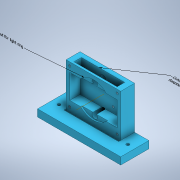
# Autodesk Inventor part: 2020PiZeroCameraLightRingMount
Saved by Autodesk Inventor 2020.2 (Build 242310000, 310)
## iProperties
Created: 2019-10-10
Part Number: 2020PiZeroCameraLightRingMount
Material: PC/ABS Plastic
Document SubType Name: Modeling
Designer: steele
Density: 0.357273 g/cm^3
Appearance: Turquoise
Author: steele
Autodesk Inventor part; units mm, degrees
ref_plane "YZ Plane" through (0, 0, 0) normal (1, 0, 0) x (0, 1, 0)
ref_plane "XZ Plane" through (0, 0, 0) normal (0, 1, 0) x (-1, 0, 0)
ref_plane "XY Plane" through (0, 0, 0) normal (0, 0, 1) x (1, 0, 0)
sketch "Sketch1" plane through (0, 0, 0) normal (0, 0, 1) x (1, 0, 0)
  line L0 (-48.5775, -37.85) -> (48.5775, -37.85)
  line L1 (48.5775, -37.85) -> (48.5775, 37.85)
  line L2 (48.5775, 37.85) -> (-48.5775, 37.85)
  line L3 (-48.5775, 37.85) -> (-48.5775, -37.85)
  line L4 (-48.5775, -37.85) -> (48.5775, 37.85) construction
  line L5 (48.5775, -37.85) -> (-48.5775, 37.85) construction
  point P0 (0, 0)
  dimension "majorPartWidth" = 97.155
  dimension "majorPartHeight" = 75.7
  constraints: 12 end point, 2 midpoint, 2 parallel, 1 horizontal, 1 perpendicular
  measures "majorPartWidth" distance of L0.start L0.end
  measures "majorPartHeight" distance of L1.end L0.end
extrude "Extrusion1" add sketch "Sketch1" against normal blind 24.725
sketch "Sketch2" plane through (0, 0, 0) normal (0, 0, 1) x (1, 0, 0)
  line L0 (-42.2275, -21.59) -> (42.2275, -21.59)
  line L1 (42.2275, -21.59) -> (42.2275, 21.59)
  line L2 (42.2275, 21.59) -> (-42.2275, 21.59)
  line L3 (-42.2275, 21.59) -> (-42.2275, -21.59)
  line L4 (-42.2275, -21.59) -> (42.2275, 21.59) construction
  line L5 (42.2275, -21.59) -> (-42.2275, 21.59) construction
  point P0 (0, 0)
  dimension "holeForPiCaseWidth" = 84.455
  dimension "holeForPiCaseHeight" = 43.18
  constraints: 12 end point, 2 midpoint, 2 parallel, 1 horizontal, 1 perpendicular
  measures "holeForPiCaseWidth" distance of L0.start L0.end
  measures "holeForPiCaseHeight" distance of L1.end L0.end
extrude "Extrusion2" cut sketch "Sketch2" against normal blind 18.375
sketch "Sketch3" plane through (0, 0, 0) normal (0, 0, 1) x (1, 0, 0)
  circle A0 centre (0, 0) radius 31.5
  circle A1 centre (0, 0) radius 18.5
  dimension "lightRingHoleExteriorDiam" = 63
  dimension "lightRingHoleInteriorDiam" = 37
  constraints: 2 centre point, 2 coincident
  measures "lightRingHoleExteriorDiam" diameter of A0
  measures "lightRingHoleInteriorDiam" diameter of A1
extrude "Extrusion3" cut sketch "Sketch3" against normal blind 2.5
sketch "Sketch4" plane through (0, 0, -2.5) normal (0, 0, 1) x (1, 0, 0)
  circle A0 centre (0, 0) radius 25.4466 construction
  circle A1 centre (0, 25.4466) radius 5
  circle A2 centre (0, -25.4466) radius 5
  dimension "holeForLightRingWires" = 10
  dimension "d13" = 10
  constraints: 3 centre point, 2 point on circle, 1 coincident
  measures "holeForLightRingWires" diameter of A1
  measures "d13" diameter of A2
extrude "Extrusion4" cut sketch "Sketch4" against normal through all
sketch "Sketch6" plane through (-48.5775, -37.85, 0) normal (0, -1, 0) x (1, 0, 0)
  line L0 (0, -24.725) -> (97.155, -24.725) projected
  line L1 (0, -24.725) -> (97.155, -24.725)
  line L2 (97.155, -24.725) -> (97.155, 25.4)
  line L3 (97.155, 25.4) -> (0, 25.4)
  line L4 (0, 25.4) -> (0, -24.725)
  point P0 (48.5775, 0)
  dimension "baseWidth" = 97.155
  dimension "baseDepth" = 50.125
  constraints: 8 end point, 2 parallel, 1 horizontal, 1 perpendicular
  measures "baseWidth" distance of L2.end L3.end
  measures "baseDepth" distance of L1.end L2.end
extrude "Extrusion6" add sketch "Sketch6" along normal blind 12.7
sketch "Sketch7" plane through (-48.5775, 37.85, 0) normal (0, 1, 0) x (1, 0, 0)
  line L0 (97.155, 0) -> (0, 0) construction
  line L1 (0, 0) -> (0, 24.725) construction
  line L2 (10.16, 3.77) -> (86.995, 3.77)
  line L3 (86.995, 3.77) -> (86.995, 17.105)
  line L4 (86.995, 17.105) -> (10.16, 17.105)
  line L5 (10.16, 17.105) -> (10.16, 3.77)
  line L6 (10.16, 3.77) -> (86.995, 17.105) construction
  line L7 (86.995, 3.77) -> (10.16, 17.105) construction
  line L8 (45.3952, 18.375) -> (45.3952, 2.5) projected
  point P0 (48.5775, 0)
  point P1 (48.5775, 10.4375)
  dimension "y" = 10.4375
  dimension "Y" = 48.5775
  dimension "piWireDepth" = 13.335
  dimension "piWireWidth" = 76.835
  constraints: 12 end point, 2 midpoint, 2 parallel, 2 perpendicular
  measures "y" distance from line of point (48.577, 10.438) L0
  measures "Y" distance from line of point (48.577, 10.438) L1
  measures "piWireDepth" distance of L4.end L2.start
  measures "piWireWidth" distance of L3.end L4.end
extrude "Extrusion7" cut sketch "Sketch7" against normal up to next
sketch "Sketch8" plane through (-48.5775, 37.85, -24.725) normal (-1, 0, 0) x (0, 0, 1)
  line L0 (24.725, -75.7) -> (24.725, 0) projected
  line L1 (24.725, -75.7) -> (28.535, -75.7)
  line L2 (28.535, -75.7) -> (28.535, -78.24)
  line L3 (28.535, -78.24) -> (24.725, -78.24)
  line L4 (24.725, -78.24) -> (24.725, -75.7)
  point P0 (24.725, -37.85)
  dimension "d30" = 3.81
  dimension "d31" = 2.54
  constraints: 8 end point, 2 parallel, 1 horizontal, 1 perpendicular
  measures "d30" distance of L2.end L3.end
  measures "d31" distance of L1.end L2.end
extrude "Extrusion8" cut sketch "Sketch8" against normal through all
sketch "Sketch9" plane through (0, 0, 0) normal (0, 0, 1) x (1, 0, 0)
  point P0 (-42.2275, 31.5)
  point P1 (42.2275, 31.5)
  point P2 (42.2275, -31.5)
  point P3 (-42.2275, -31.5)
hole "Hole1" at (-42.2275, 31.5, 0) at (42.2275, 31.5, 0) at (42.2275, -31.5, 0) at (-42.2275, -31.5, 0) direction (0, 0, -1) diameter 3.9624 depth 14.986 tip angle 120 thread size "10-32 UNF" class "2B" standard "ANSI Unified Screw Threads"
sketch "Sketch10" plane through (0, 0, -24.725) normal (0, 0, -1) x (-1, 0, 0)
  point P0 (-39.0525, 23.7022)
  point P1 (-16.8275, 23.7022)
  point P2 (-16.8275, -11.2228)
  point P3 (-39.0525, -11.2228)
hole "Hole3" at (39.0525, 23.7022, -24.725) at (16.8275, 23.7022, -24.725) at (16.8275, -11.2228, -24.725) at (39.0525, -11.2228, -24.725) direction (0, 0, 1) diameter 3.9624 depth 11.9507 tip angle 120 thread size "10-32 UNF" class "2B" standard "ANSI Unified Screw Threads"
sketch "Sketch11" plane through (48.5775, 37.85, 0) normal (1, 0, 0) x (0, 0, -1)
  line L0 (-25.4, -75.7) -> (-25.4, -88.4) projected
  line L1 (24.725, 0) -> (24.725, -88.4) projected
  line L2 (-25.4, -88.4) -> (24.725, -88.4)
  line L3 (24.725, -88.4) -> (24.725, -75.7)
  line L4 (24.725, -75.7) -> (-25.4, -75.7)
  line L5 (-25.4, -75.7) -> (-25.4, -88.4)
  point P0 (0, -37.85)
  dimension "d50" = 12.7
  constraints: 8 end point, 2 parallel, 1 horizontal, 1 perpendicular, 1 point on line
  measures "d50" distance of L3.end L2.end
extrude "Extrusion9" add sketch "Sketch11" along normal blind 25.4
sketch "Sketch12" plane through (-48.5775, 37.85, -24.725) normal (-1, 0, 0) x (0, 0, 1)
  line L0 (50.125, -75.7) -> (50.125, -88.4) projected
  line L1 (50.125, -88.4) -> (0, -88.4) projected
  line L2 (50.125, -75.7) -> (0, -75.7)
  line L3 (0, -75.7) -> (0, -88.4)
  line L4 (0, -88.4) -> (50.125, -88.4)
  line L5 (50.125, -88.4) -> (50.125, -75.7)
  point P0 (24.725, -37.85)
  constraints: 8 end point, 2 parallel, 1 horizontal, 1 perpendicular
extrude "Extrusion10" add sketch "Sketch12" along normal blind 25.4
sketch "Sketch13" plane through (-48.5775, -37.85, 0) normal (0, 1, 0) x (1, 0, 0)
  line L0 (97.155, 0) -> (0, 0) projected
  line L1 (0, 0) -> (0, 24.725) projected
  line L2 (97.155, 0) -> (97.155, 24.725) projected
  point P0 (48.5775, 0)
  point P1 (109.855, 0)
  point P2 (-12.7, 0)
  dimension "d62" = 0
  dimension "d63" = 0
  dimension "d64" = 12.7
  dimension "d65" = 12.7
  measures "d62" distance from line of point (-12.7, 0) L0
  measures "d63" distance from line of L0 point (109.855, 0)
  measures "d64" distance from line of point (-12.7, 0) L1
  measures "d65" distance from line of point (109.855, 0) L2
hole "Hole5" at (61.2775, -37.85, 0) at (-61.2775, -37.85, 0) direction (0, -1, 0) diameter 5.1054 end through all clearance for "Socket Head Cap Screw" size "#10" standard "Ansi Unified Screw Threads"
sketch "Sketch14" plane through (-48.5775, -50.55, 0) normal (0, -1, 0) x (1, 0, 0)
  circle A0 centre (-12.7, 0) radius 2.5527 construction
  circle A1 centre (109.855, 0) radius 2.5527 construction
  line L0 (-12.7, 0) -> (109.855, 0) construction
  spline S0 degree 2 poles (30.5129, 11.4249) (30.5129, 10.5552) (29.8079, 9.1555) (29.2162, 8.7644) knots 0 0 0 1 2 2 2
  spline S1 degree 2 poles (29.2162, 8.7644) (28.7325, 8.4608) (27.7393, 8.255) (26.9674, 8.255) knots 0 0 0 1 2 2 2
  line L1 (26.9674, 8.255) -> (25.506, 8.255)
  line L2 (25.506, 8.255) -> (25.506, 14.605)
  line L3 (25.506, 14.605) -> (26.952, 14.605)
  spline S2 degree 2 poles (26.952, 14.605) (27.8474, 14.605) (28.8663, 14.3374) (29.2265, 14.1007) knots 0 0 0 1 2 2 2
  spline S3 degree 2 poles (29.2265, 14.1007) (29.8388, 13.6942) (30.5129, 12.3511) (30.5129, 11.4249) knots 0 0 0 1 2 2 2
  spline S4 degree 2 poles (29.633, 11.4351) (29.633, 12.1659) (29.1493, 13.2002) (28.6707, 13.4935) knots 0 0 0 1 2 2 2
  spline S5 degree 2 poles (28.6707, 13.4935) (28.3311, 13.6942) (27.5644, 13.8743) (26.9932, 13.8743) knots 0 0 0 1 2 2 2
  line L4 (26.9932, 13.8743) -> (26.3499, 13.8743)
  line L5 (26.3499, 13.8743) -> (26.3499, 8.9857)
  line L6 (26.3499, 8.9857) -> (26.9932, 8.9857)
  spline S6 degree 2 poles (26.9932, 8.9857) (27.5541, 8.9857) (28.4031, 9.1658) (28.7479, 9.4077) knots 0 0 0 1 2 2 2
  spline S7 degree 2 poles (28.7479, 9.4077) (29.1904, 9.7061) (29.633, 10.6941) (29.633, 11.4351) knots 0 0 0 1 2 2 2
  spline S8 degree 2 poles (33.4358, 8.1469) (32.2934, 8.1469) (31.0378, 9.4283) (31.0378, 10.6118) knots 0 0 0 1 2 2 2
  spline S9 degree 2 poles (31.0378, 10.6118) (31.0378, 11.7748) (32.2574, 13.1539) (33.2402, 13.1539) knots 0 0 0 1 2 2 2
  spline S10 degree 2 poles (33.2402, 13.1539) (33.6828, 13.1539) (34.3672, 12.8966) (34.6193, 12.6238) knots 0 0 0 1 2 2 2
  spline S11 degree 2 poles (34.6193, 12.6238) (34.8766, 12.3511) (35.1494, 11.5638) (35.1494, 10.9926) knots 0 0 0 1 2 2 2
  line L7 (35.1494, 10.9926) -> (35.1494, 10.5552)
  line L8 (35.1494, 10.5552) -> (31.8509, 10.5552)
  spline S12 degree 2 poles (31.8509, 10.5552) (31.8509, 9.7267) (32.6845, 8.8468) (33.4255, 8.8468) knots 0 0 0 1 2 2 2
  spline S13 degree 2 poles (33.4255, 8.8468) (33.6879, 8.8468) (34.1974, 8.9651) (34.4032, 9.0578) knots 0 0 0 1 2 2 2
  spline S14 degree 2 poles (34.4032, 9.0578) (34.6193, 9.1607) (34.9178, 9.3408) (35.0156, 9.4231) knots 0 0 0 1 2 2 2
  line L9 (35.0156, 9.4231) -> (35.0619, 9.4231)
  line L10 (35.0619, 9.4231) -> (35.0619, 8.5483)
  spline S15 degree 2 poles (35.0619, 8.5483) (34.9229, 8.4917) (34.501, 8.327) (34.3363, 8.2807) knots 0 0 0 1 2 2 2
  spline S16 degree 2 poles (34.3363, 8.2807) (34.1047, 8.2138) (33.724, 8.1469) (33.4358, 8.1469) knots 0 0 0 1 2 2 2
  spline S17 degree 2 poles (34.3672, 11.1676) (34.3569, 11.4918) (34.2231, 11.9652) (34.0945, 12.1247) knots 0 0 0 1 2 2 2
  spline S18 degree 2 poles (34.0945, 12.1247) (33.9555, 12.3048) (33.5181, 12.4952) (33.1939, 12.4952) knots 0 0 0 1 2 2 2
  spline S19 degree 2 poles (33.1939, 12.4952) (32.8749, 12.4952) (32.4272, 12.3048) (32.2419, 12.1195) knots 0 0 0 1 2 2 2
  spline S20 degree 2 poles (32.2419, 12.1195) (32.0618, 11.9291) (31.8766, 11.4712) (31.8509, 11.1676) knots 0 0 0 1 2 2 2
  line L11 (31.8509, 11.1676) -> (34.3672, 11.1676)
  spline S21 degree 2 poles (37.2489, 8.1418) (36.7703, 8.1418) (35.9418, 8.3991) (35.6691, 8.5432) knots 0 0 0 1 2 2 2
  line L12 (35.6691, 8.5432) -> (35.6691, 9.4437)
  line L13 (35.6691, 9.4437) -> (35.7103, 9.4437)
  spline S22 degree 2 poles (35.7103, 9.4437) (35.8132, 9.3614) (36.0911, 9.1658) (36.3226, 9.0578) knots 0 0 0 1 2 2 2
  spline S23 degree 2 poles (36.3226, 9.0578) (36.5233, 8.96) (37.0173, 8.8159) (37.2797, 8.8159) knots 0 0 0 1 2 2 2
  spline S24 degree 2 poles (37.2797, 8.8159) (37.4701, 8.8159) (37.9075, 8.9034) (38.0105, 8.9754) knots 0 0 0 1 2 2 2
  spline S25 degree 2 poles (38.0105, 8.9754) (38.1597, 9.0732) (38.2935, 9.2945) (38.2935, 9.5209) knots 0 0 0 1 2 2 2
  spline S26 degree 2 poles (38.2935, 9.5209) (38.2935, 9.8039) (37.9847, 10.0972) (37.5885, 10.195) knots 0 0 0 1 2 2 2
  spline S27 degree 2 poles (37.5885, 10.195) (37.4341, 10.231) (36.9401, 10.3339) (36.7291, 10.3905) knots 0 0 0 1 2 2 2
  spline S28 degree 2 poles (36.7291, 10.3905) (36.1837, 10.5501) (35.6897, 11.2087) (35.6897, 11.677) knots 0 0 0 1 2 2 2
  spline S29 degree 2 poles (35.6897, 11.677) (35.6897, 12.3254) (36.6622, 13.1333) (37.465, 13.1333) knots 0 0 0 1 2 2 2
  spline S30 degree 2 poles (37.465, 13.1333) (37.8612, 13.1333) (38.664, 12.9377) (38.9367, 12.7885) knots 0 0 0 1 2 2 2
  line L14 (38.9367, 12.7885) -> (38.9367, 11.9291)
  line L15 (38.9367, 11.9291) -> (38.8956, 11.9291)
  spline S31 degree 2 poles (38.8956, 11.9291) (38.5868, 12.1762) (37.8355, 12.4592) (37.4496, 12.4592) knots 0 0 0 1 2 2 2
  spline S32 degree 2 poles (37.4496, 12.4592) (37.0533, 12.4592) (36.5079, 12.1247) (36.5079, 11.7902) knots 0 0 0 1 2 2 2
  spline S33 degree 2 poles (36.5079, 11.7902) (36.5079, 11.4866) (36.8321, 11.1933) (37.1923, 11.1007) knots 0 0 0 1 2 2 2
  spline S34 degree 2 poles (37.1923, 11.1007) (37.3672, 11.0544) (37.8098, 10.9617) (38.0516, 10.9051) knots 0 0 0 1 2 2 2
  spline S35 degree 2 poles (38.0516, 10.9051) (38.5765, 10.7713) (39.1117, 10.159) (39.1117, 9.6289) knots 0 0 0 1 2 2 2
  spline S36 degree 2 poles (39.1117, 9.6289) (39.1117, 9.3202) (38.8698, 8.7747) (38.6331, 8.574) knots 0 0 0 1 2 2 2
  spline S37 degree 2 poles (38.6331, 8.574) (38.381, 8.3631) (37.7377, 8.1418) (37.2489, 8.1418) knots 0 0 0 1 2 2 2
  line L16 (40.676, 8.255) -> (39.8733, 8.255)
  line L17 (39.8733, 8.255) -> (39.8733, 13.0201)
  line L18 (39.8733, 13.0201) -> (40.676, 13.0201)
  line L19 (40.676, 13.0201) -> (40.676, 8.255)
  line L20 (40.7326, 13.8125) -> (39.8218, 13.8125)
  line L21 (39.8218, 13.8125) -> (39.8218, 14.6462)
  line L22 (39.8218, 14.6462) -> (40.7326, 14.6462)
  line L23 (40.7326, 14.6462) -> (40.7326, 13.8125)
  spline S38 degree 2 poles (42.0242, 7.4934) (42.1066, 7.4574) (42.4205, 7.3442) (42.6212, 7.2979) knots 0 0 0 1 2 2 2
  spline S39 degree 2 poles (42.6212, 7.2979) (42.8424, 7.2413) (43.2181, 7.1744) (43.4394, 7.1744) knots 0 0 0 1 2 2 2
  spline S40 degree 2 poles (43.4394, 7.1744) (43.8099, 7.1744) (44.3244, 7.3699) (44.4685, 7.5449) knots 0 0 0 1 2 2 2
  spline S41 degree 2 poles (44.4685, 7.5449) (44.6075, 7.7198) (44.7155, 8.1778) (44.7155, 8.4711) knots 0 0 0 1 2 2 2
  line L24 (44.7155, 8.4711) -> (44.7155, 8.8879)
  spline S42 degree 2 poles (44.7155, 8.8879) (44.3913, 8.6049) (43.7687, 8.3373) (43.3004, 8.3373) knots 0 0 0 1 2 2 2
  spline S43 degree 2 poles (43.3004, 8.3373) (42.4874, 8.3373) (41.5251, 9.5466) (41.5251, 10.6838) knots 0 0 0 1 2 2 2
  spline S44 degree 2 poles (41.5251, 10.6838) (41.5251, 11.2756) (41.8596, 12.1916) (42.1374, 12.5158) knots 0 0 0 1 2 2 2
  spline S45 degree 2 poles (42.1374, 12.5158) (42.405, 12.8194) (43.1409, 13.1539) (43.532, 13.1539) knots 0 0 0 1 2 2 2
  spline S46 degree 2 poles (43.532, 13.1539) (43.9025, 13.1539) (44.4428, 12.9789) (44.7155, 12.8194) knots 0 0 0 1 2 2 2
  line L25 (44.7155, 12.8194) -> (44.7618, 13.0201)
  line L26 (44.7618, 13.0201) -> (45.5183, 13.0201)
  line L27 (45.5183, 13.0201) -> (45.5183, 8.8005)
  spline S47 degree 2 poles (45.5183, 8.8005) (45.5183, 7.586) (44.4634, 6.4539) (43.3776, 6.4539) knots 0 0 0 1 2 2 2
  spline S48 degree 2 poles (43.3776, 6.4539) (43.0277, 6.4539) (42.297, 6.5672) (41.9831, 6.6598) knots 0 0 0 1 2 2 2
  line L28 (41.9831, 6.6598) -> (41.9831, 7.4934)
  line L29 (41.9831, 7.4934) -> (42.0242, 7.4934)
  line L30 (44.7155, 9.5466) -> (44.7155, 12.1659)
  spline S49 degree 2 poles (44.7155, 12.1659) (44.4171, 12.3099) (43.9128, 12.4334) (43.6606, 12.4334) knots 0 0 0 1 2 2 2
  spline S50 degree 2 poles (43.6606, 12.4334) (43.0534, 12.4334) (42.3536, 11.5381) (42.3536, 10.6993) knots 0 0 0 1 2 2 2
  spline S51 degree 2 poles (42.3536, 10.6993) (42.3536, 9.9068) (42.8836, 9.0783) (43.4805, 9.0783) knots 0 0 0 1 2 2 2
  spline S52 degree 2 poles (43.4805, 9.0783) (43.7944, 9.0783) (44.4531, 9.3253) (44.7155, 9.5466) knots 0 0 0 1 2 2 2
  line L31 (50.4223, 8.255) -> (49.6195, 8.255)
  line L32 (49.6195, 8.255) -> (49.6195, 10.972)
  spline S53 degree 2 poles (49.6195, 10.972) (49.6195, 11.3014) (49.5578, 11.8674) (49.4652, 12.0372) knots 0 0 0 1 2 2 2
  spline S54 degree 2 poles (49.4652, 12.0372) (49.3674, 12.2173) (49.0175, 12.3923) (48.719, 12.3923) knots 0 0 0 1 2 2 2
  spline S55 degree 2 poles (48.719, 12.3923) (48.4206, 12.3923) (47.7876, 12.0732) (47.484, 11.8159) knots 0 0 0 1 2 2 2
  line L33 (47.484, 11.8159) -> (47.484, 8.255)
  line L34 (47.484, 8.255) -> (46.6812, 8.255)
  line L35 (46.6812, 8.255) -> (46.6812, 13.0201)
  line L36 (46.6812, 13.0201) -> (47.484, 13.0201)
  line L37 (47.484, 13.0201) -> (47.484, 12.49)
  spline S56 degree 2 poles (47.484, 12.49) (47.8442, 12.8142) (48.5389, 13.1539) (48.93, 13.1539) knots 0 0 0 1 2 2 2
  spline S57 degree 2 poles (48.93, 13.1539) (49.6298, 13.1539) (50.4223, 12.2276) (50.4223, 11.3477) knots 0 0 0 1 2 2 2
  line L38 (50.4223, 11.3477) -> (50.4223, 8.255)
  spline S58 degree 2 poles (53.6179, 8.1469) (52.4755, 8.1469) (51.2199, 9.4283) (51.2199, 10.6118) knots 0 0 0 1 2 2 2
  spline S59 degree 2 poles (51.2199, 10.6118) (51.2199, 11.7748) (52.4395, 13.1539) (53.4223, 13.1539) knots 0 0 0 1 2 2 2
  spline S60 degree 2 poles (53.4223, 13.1539) (53.8649, 13.1539) (54.5493, 12.8966) (54.8014, 12.6238) knots 0 0 0 1 2 2 2
  spline S61 degree 2 poles (54.8014, 12.6238) (55.0587, 12.3511) (55.3314, 11.5638) (55.3314, 10.9926) knots 0 0 0 1 2 2 2
  line L39 (55.3314, 10.9926) -> (55.3314, 10.5552)
  line L40 (55.3314, 10.5552) -> (52.0329, 10.5552)
  spline S62 degree 2 poles (52.0329, 10.5552) (52.0329, 9.7267) (52.8666, 8.8468) (53.6076, 8.8468) knots 0 0 0 1 2 2 2
  spline S63 degree 2 poles (53.6076, 8.8468) (53.87, 8.8468) (54.3795, 8.9651) (54.5853, 9.0578) knots 0 0 0 1 2 2 2
  spline S64 degree 2 poles (54.5853, 9.0578) (54.8014, 9.1607) (55.0999, 9.3408) (55.1977, 9.4231) knots 0 0 0 1 2 2 2
  line L41 (55.1977, 9.4231) -> (55.244, 9.4231)
  line L42 (55.244, 9.4231) -> (55.244, 8.5483)
  spline S65 degree 2 poles (55.244, 8.5483) (55.105, 8.4917) (54.6831, 8.327) (54.5184, 8.2807) knots 0 0 0 1 2 2 2
  spline S66 degree 2 poles (54.5184, 8.2807) (54.2868, 8.2138) (53.906, 8.1469) (53.6179, 8.1469) knots 0 0 0 1 2 2 2
  spline S67 degree 2 poles (54.5493, 11.1676) (54.539, 11.4918) (54.4052, 11.9652) (54.2765, 12.1247) knots 0 0 0 1 2 2 2
  spline S68 degree 2 poles (54.2765, 12.1247) (54.1376, 12.3048) (53.7002, 12.4952) (53.376, 12.4952) knots 0 0 0 1 2 2 2
  spline S69 degree 2 poles (53.376, 12.4952) (53.057, 12.4952) (52.6093, 12.3048) (52.424, 12.1195) knots 0 0 0 1 2 2 2
  spline S70 degree 2 poles (52.424, 12.1195) (52.2439, 11.9291) (52.0587, 11.4712) (52.0329, 11.1676) knots 0 0 0 1 2 2 2
  line L43 (52.0329, 11.1676) -> (54.5493, 11.1676)
  line L44 (59.8084, 8.255) -> (59.0056, 8.255)
  line L45 (59.0056, 8.255) -> (59.0056, 8.7387)
  spline S71 degree 2 poles (59.0056, 8.7387) (58.8203, 8.5843) (58.5476, 8.3785) (58.3624, 8.291) knots 0 0 0 1 2 2 2
  spline S72 degree 2 poles (58.3624, 8.291) (58.1926, 8.2087) (57.8272, 8.1212) (57.5853, 8.1212) knots 0 0 0 1 2 2 2
  spline S73 degree 2 poles (57.5853, 8.1212) (57.1943, 8.1212) (56.5356, 8.4454) (56.304, 8.7593) knots 0 0 0 1 2 2 2
  spline S74 degree 2 poles (56.304, 8.7593) (56.0725, 9.0732) (55.8152, 9.9994) (55.8152, 10.6015) knots 0 0 0 1 2 2 2
  spline S75 degree 2 poles (55.8152, 10.6015) (55.8152, 11.2293) (56.1394, 12.1453) (56.4224, 12.49) knots 0 0 0 1 2 2 2
  spline S76 degree 2 poles (56.4224, 12.49) (56.6848, 12.7988) (57.4207, 13.1539) (57.8272, 13.1539) knots 0 0 0 1 2 2 2
  spline S77 degree 2 poles (57.8272, 13.1539) (58.1823, 13.1539) (58.7123, 12.9943) (59.0056, 12.8297) knots 0 0 0 1 2 2 2
  line L46 (59.0056, 12.8297) -> (59.0056, 14.888)
  line L47 (59.0056, 14.888) -> (59.8084, 14.888)
  line L48 (59.8084, 14.888) -> (59.8084, 8.255)
  line L49 (59.0056, 9.4128) -> (59.0056, 12.1659)
  spline S78 degree 2 poles (59.0056, 12.1659) (58.7071, 12.3099) (58.2337, 12.418) (57.961, 12.418) knots 0 0 0 1 2 2 2
  spline S79 degree 2 poles (57.961, 12.418) (57.3435, 12.418) (56.6436, 11.4918) (56.6436, 10.617) knots 0 0 0 1 2 2 2
  spline S80 degree 2 poles (56.6436, 10.617) (56.6436, 9.773) (57.1788, 8.8828) (57.7706, 8.8828) knots 0 0 0 1 2 2 2
  spline S81 degree 2 poles (57.7706, 8.8828) (58.0845, 8.8828) (58.7226, 9.171) (59.0056, 9.4128) knots 0 0 0 1 2 2 2
  spline S82 degree 2 poles (67.6918, 10.7147) (67.6918, 9.5466) (66.5597, 8.1212) (65.7055, 8.1212) knots 0 0 0 1 2 2 2
  spline S83 degree 2 poles (65.7055, 8.1212) (65.3196, 8.1212) (64.769, 8.3116) (64.5014, 8.4763) knots 0 0 0 1 2 2 2
  line L50 (64.5014, 8.4763) -> (64.4499, 8.255)
  line L51 (64.4499, 8.255) -> (63.6986, 8.255)
  line L52 (63.6986, 8.255) -> (63.6986, 14.888)
  line L53 (63.6986, 14.888) -> (64.5014, 14.888)
  line L54 (64.5014, 14.888) -> (64.5014, 12.5209)
  spline S84 degree 2 poles (64.5014, 12.5209) (64.805, 12.7937) (65.51, 13.1539) (65.9577, 13.1539) knots 0 0 0 1 2 2 2
  spline S85 degree 2 poles (65.9577, 13.1539) (66.7656, 13.1539) (67.6918, 11.8623) (67.6918, 10.7147) knots 0 0 0 1 2 2 2
  spline S86 degree 2 poles (66.8633, 10.653) (66.8633, 11.5072) (66.3436, 12.3923) (65.7673, 12.3923) knots 0 0 0 1 2 2 2
  spline S87 degree 2 poles (65.7673, 12.3923) (65.4431, 12.3923) (64.7741, 12.0835) (64.5014, 11.8468) knots 0 0 0 1 2 2 2
  line L55 (64.5014, 11.8468) -> (64.5014, 9.1144)
  spline S88 degree 2 poles (64.5014, 9.1144) (64.805, 8.9651) (65.2733, 8.8416) (65.5511, 8.8416) knots 0 0 0 1 2 2 2
  spline S89 degree 2 poles (65.5511, 8.8416) (66.1635, 8.8416) (66.8633, 9.7113) (66.8633, 10.653) knots 0 0 0 1 2 2 2
  line L56 (72.2665, 13.0201) -> (69.7039, 6.5003)
  line L57 (69.7039, 6.5003) -> (68.8445, 6.5003)
  line L58 (68.8445, 6.5003) -> (69.6987, 8.4866)
  line L59 (69.6987, 8.4866) -> (67.9697, 13.0201)
  line L60 (67.9697, 13.0201) -> (68.8342, 13.0201)
  line L61 (68.8342, 13.0201) -> (70.1361, 9.49)
  line L62 (70.1361, 9.49) -> (71.4329, 13.0201)
  line L63 (71.4329, 13.0201) -> (72.2665, 13.0201)
  line L64 (33.495, -2.3804) -> (32.3989, -2.3804)
  line L65 (32.3989, -2.3804) -> (30.392, 0.1463)
  line L66 (30.392, 0.1463) -> (29.4246, 0.1463)
  line L67 (29.4246, 0.1463) -> (29.4246, -2.3804)
  line L68 (29.4246, -2.3804) -> (28.5807, -2.3804)
  line L69 (28.5807, -2.3804) -> (28.5807, 3.9696)
  line L70 (28.5807, 3.9696) -> (30.217, 3.9696)
  spline S90 degree 2 poles (30.217, 3.9696) (30.7625, 3.9696) (31.4984, 3.8513) (31.8328, 3.6352) knots 0 0 0 1 2 2 2
  spline S91 degree 2 poles (31.8328, 3.6352) (32.1673, 3.419) (32.5533, 2.7449) (32.5533, 2.2458) knots 0 0 0 1 2 2 2
  spline S92 degree 2 poles (32.5533, 2.2458) (32.5533, 1.5511) (31.8431, 0.6094) (31.2359, 0.383) knots 0 0 0 1 2 2 2
  line L71 (31.2359, 0.383) -> (33.495, -2.3804)
  spline S93 degree 2 poles (31.6733, 2.1789) (31.6733, 2.4568) (31.4778, 2.8839) (31.2719, 3.0228) knots 0 0 0 1 2 2 2
  spline S94 degree 2 poles (31.2719, 3.0228) (31.0918, 3.1412) (30.6133, 3.2389) (30.2634, 3.2389) knots 0 0 0 1 2 2 2
  line L72 (30.2634, 3.2389) -> (29.4246, 3.2389)
  line L73 (29.4246, 3.2389) -> (29.4246, 0.8512)
  line L74 (29.4246, 0.8512) -> (30.1656, 0.8512)
  spline S95 degree 2 poles (30.1656, 0.8512) (30.5309, 0.8512) (31.1124, 0.9799) (31.3131, 1.1806) knots 0 0 0 1 2 2 2
  spline S96 degree 2 poles (31.3131, 1.1806) (31.4984, 1.3555) (31.6733, 1.8495) (31.6733, 2.1789) knots 0 0 0 1 2 2 2
  spline S97 degree 2 poles (37.8535, 0.0022) (37.8535, -1.202) (36.6957, -2.5142) (35.7283, -2.5142) knots 0 0 0 1 2 2 2
  spline S98 degree 2 poles (35.7283, -2.5142) (34.7351, -2.5142) (33.5979, -1.1608) (33.5979, 0.0022) knots 0 0 0 1 2 2 2
  spline S99 degree 2 poles (33.5979, 0.0022) (33.5979, 1.196) (34.7711, 2.5185) (35.7283, 2.5185) knots 0 0 0 1 2 2 2
  spline S100 degree 2 poles (35.7283, 2.5185) (36.6957, 2.5185) (37.8535, 1.2012) (37.8535, 0.0022) knots 0 0 0 1 2 2 2
  spline S101 degree 2 poles (37.025, 0.0022) (37.025, 0.9284) (36.3509, 1.829) (35.7283, 1.829) knots 0 0 0 1 2 2 2
  spline S102 degree 2 poles (35.7283, 1.829) (35.1056, 1.829) (34.4264, 0.9284) (34.4264, 0.0022) knots 0 0 0 1 2 2 2
  spline S103 degree 2 poles (34.4264, 0.0022) (34.4264, -0.8984) (35.1056, -1.8246) (35.7283, -1.8246) knots 0 0 0 1 2 2 2
  spline S104 degree 2 poles (35.7283, -1.8246) (36.3458, -1.8246) (37.025, -0.9138) (37.025, 0.0022) knots 0 0 0 1 2 2 2
  spline S105 degree 2 poles (42.67, 0.0794) (42.67, -1.0887) (41.538, -2.5142) (40.6837, -2.5142) knots 0 0 0 1 2 2 2
  spline S106 degree 2 poles (40.6837, -2.5142) (40.2978, -2.5142) (39.7472, -2.3238) (39.4796, -2.1591) knots 0 0 0 1 2 2 2
  line L75 (39.4796, -2.1591) -> (39.4281, -2.3804)
  line L76 (39.4281, -2.3804) -> (38.6769, -2.3804)
  line L77 (38.6769, -2.3804) -> (38.6769, 4.2527)
  line L78 (38.6769, 4.2527) -> (39.4796, 4.2527)
  line L79 (39.4796, 4.2527) -> (39.4796, 1.8856)
  spline S107 degree 2 poles (39.4796, 1.8856) (39.7832, 2.1583) (40.4882, 2.5185) (40.9359, 2.5185) knots 0 0 0 1 2 2 2
  spline S108 degree 2 poles (40.9359, 2.5185) (41.7438, 2.5185) (42.67, 1.2269) (42.67, 0.0794) knots 0 0 0 1 2 2 2
  spline S109 degree 2 poles (41.8416, 0.0176) (41.8416, 0.8718) (41.3218, 1.7569) (40.7455, 1.7569) knots 0 0 0 1 2 2 2
  spline S110 degree 2 poles (40.7455, 1.7569) (40.4213, 1.7569) (39.7523, 1.4482) (39.4796, 1.2115) knots 0 0 0 1 2 2 2
  line L80 (39.4796, 1.2115) -> (39.4796, -1.521)
  spline S111 degree 2 poles (39.4796, -1.521) (39.7832, -1.6702) (40.2515, -1.7937) (40.5294, -1.7937) knots 0 0 0 1 2 2 2
  spline S112 degree 2 poles (40.5294, -1.7937) (41.1417, -1.7937) (41.8416, -0.9241) (41.8416, 0.0176) knots 0 0 0 1 2 2 2
  spline S113 degree 2 poles (48.0629, -2.4936) (47.3734, -2.4936) (46.4059, -2.2054) (45.9788, -1.9996) knots 0 0 0 1 2 2 2
  line L81 (45.9788, -1.9996) -> (45.9788, -0.9395)
  line L82 (45.9788, -0.9395) -> (46.0406, -0.9395)
  spline S114 degree 2 poles (46.0406, -0.9395) (46.4574, -1.3306) (47.5123, -1.7629) (48.0012, -1.7629) knots 0 0 0 1 2 2 2
  spline S115 degree 2 poles (48.0012, -1.7629) (48.701, -1.7629) (49.4163, -1.1814) (49.4163, -0.7028) knots 0 0 0 1 2 2 2
  spline S116 degree 2 poles (49.4163, -0.7028) (49.4163, -0.322) (49.0406, 0.1514) (48.6341, 0.2698) knots 0 0 0 1 2 2 2
  spline S117 degree 2 poles (48.6341, 0.2698) (48.3408, 0.3521) (47.8519, 0.4653) (47.4866, 0.5579) knots 0 0 0 1 2 2 2
  spline S118 degree 2 poles (47.4866, 0.5579) (47.1572, 0.6454) (46.6375, 0.9078) (46.4368, 1.1188) knots 0 0 0 1 2 2 2
  spline S119 degree 2 poles (46.4368, 1.1188) (46.2413, 1.3298) (46.0251, 1.8959) (46.0251, 2.2664) knots 0 0 0 1 2 2 2
  spline S120 degree 2 poles (46.0251, 2.2664) (46.0251, 3.0382) (47.2293, 4.0828) (48.1607, 4.0828) knots 0 0 0 1 2 2 2
  spline S121 degree 2 poles (48.1607, 4.0828) (48.6959, 4.0828) (49.6427, 3.8719) (50.0492, 3.6712) knots 0 0 0 1 2 2 2
  line L83 (50.0492, 3.6712) -> (50.0492, 2.6626)
  line L84 (50.0492, 2.6626) -> (49.9875, 2.6626)
  spline S122 degree 2 poles (49.9875, 2.6626) (49.6839, 2.9405) (48.737, 3.3521) (48.2173, 3.3521) knots 0 0 0 1 2 2 2
  spline S123 degree 2 poles (48.2173, 3.3521) (47.6307, 3.3521) (46.9051, 2.8015) (46.9051, 2.3538) knots 0 0 0 1 2 2 2
  spline S124 degree 2 poles (46.9051, 2.3538) (46.9051, 1.9525) (47.3322, 1.4739) (47.7336, 1.3658) knots 0 0 0 1 2 2 2
  spline S125 degree 2 poles (47.7336, 1.3658) (48.0012, 1.2938) (48.7782, 1.1085) (49.0355, 1.0313) knots 0 0 0 1 2 2 2
  spline S126 degree 2 poles (49.0355, 1.0313) (49.689, 0.8307) (50.2962, 0.0228) (50.2962, -0.569) knots 0 0 0 1 2 2 2
  spline S127 degree 2 poles (50.2962, -0.569) (50.2962, -0.9447) (49.9926, -1.6651) (49.7199, -1.9172) knots 0 0 0 1 2 2 2
  spline S128 degree 2 poles (49.7199, -1.9172) (49.4163, -2.1951) (48.6444, -2.4936) (48.0629, -2.4936) knots 0 0 0 1 2 2 2
  spline S129 degree 2 poles (52.5347, -2.473) (51.8811, -2.473) (51.1453, -1.7268) (51.1453, -0.9189) knots 0 0 0 1 2 2 2
  line L85 (51.1453, -0.9189) -> (51.1453, 1.7209)
  line L86 (51.1453, 1.7209) -> (50.605, 1.7209)
  line L87 (50.605, 1.7209) -> (50.605, 2.3847)
  line L88 (50.605, 2.3847) -> (51.1453, 2.3847)
  line L89 (51.1453, 2.3847) -> (51.1453, 3.7535)
  line L90 (51.1453, 3.7535) -> (51.948, 3.7535)
  line L91 (51.948, 3.7535) -> (51.948, 2.3847)
  line L92 (51.948, 2.3847) -> (53.4249, 2.3847)
  line L93 (53.4249, 2.3847) -> (53.4249, 1.7209)
  line L94 (53.4249, 1.7209) -> (51.948, 1.7209)
  line L95 (51.948, 1.7209) -> (51.948, -0.5484)
  spline S130 degree 2 poles (51.948, -0.5484) (51.948, -0.9086) (51.9738, -1.3049) (52.0613, -1.4747) knots 0 0 0 1 2 2 2
  spline S131 degree 2 poles (52.0613, -1.4747) (52.1333, -1.6239) (52.4575, -1.7731) (52.7354, -1.7731) knots 0 0 0 1 2 2 2
  spline S132 degree 2 poles (52.7354, -1.7731) (52.9309, -1.7731) (53.2963, -1.6548) (53.3786, -1.6188) knots 0 0 0 1 2 2 2
  line L96 (53.3786, -1.6188) -> (53.4249, -1.6188)
  line L97 (53.4249, -1.6188) -> (53.4249, -2.3392)
  spline S133 degree 2 poles (53.4249, -2.3392) (53.1985, -2.4009) (52.7354, -2.473) (52.5347, -2.473) knots 0 0 0 1 2 2 2
  spline S134 degree 2 poles (56.0853, -2.4884) (54.9429, -2.4884) (53.6873, -1.2071) (53.6873, -0.0236) knots 0 0 0 1 2 2 2
  spline S135 degree 2 poles (53.6873, -0.0236) (53.6873, 1.1394) (54.9069, 2.5185) (55.8898, 2.5185) knots 0 0 0 1 2 2 2
  spline S136 degree 2 poles (55.8898, 2.5185) (56.3323, 2.5185) (57.0167, 2.2612) (57.2689, 1.9885) knots 0 0 0 1 2 2 2
  spline S137 degree 2 poles (57.2689, 1.9885) (57.5262, 1.7157) (57.7989, 0.9284) (57.7989, 0.3572) knots 0 0 0 1 2 2 2
  line L98 (57.7989, 0.3572) -> (57.7989, -0.0802)
  line L99 (57.7989, -0.0802) -> (54.5004, -0.0802)
  spline S138 degree 2 poles (54.5004, -0.0802) (54.5004, -0.9086) (55.334, -1.7886) (56.075, -1.7886) knots 0 0 0 1 2 2 2
  spline S139 degree 2 poles (56.075, -1.7886) (56.3375, -1.7886) (56.8469, -1.6702) (57.0527, -1.5776) knots 0 0 0 1 2 2 2
  spline S140 degree 2 poles (57.0527, -1.5776) (57.2689, -1.4747) (57.5673, -1.2946) (57.6651, -1.2122) knots 0 0 0 1 2 2 2
  line L100 (57.6651, -1.2122) -> (57.7114, -1.2122)
  line L101 (57.7114, -1.2122) -> (57.7114, -2.087)
  spline S141 degree 2 poles (57.7114, -2.087) (57.5725, -2.1437) (57.1505, -2.3083) (56.9858, -2.3546) knots 0 0 0 1 2 2 2
  spline S142 degree 2 poles (56.9858, -2.3546) (56.7543, -2.4215) (56.3735, -2.4884) (56.0853, -2.4884) knots 0 0 0 1 2 2 2
  spline S143 degree 2 poles (57.0167, 0.5322) (57.0064, 0.8564) (56.8726, 1.3298) (56.744, 1.4893) knots 0 0 0 1 2 2 2
  spline S144 degree 2 poles (56.744, 1.4893) (56.6051, 1.6694) (56.1677, 1.8598) (55.8435, 1.8598) knots 0 0 0 1 2 2 2
  spline S145 degree 2 poles (55.8435, 1.8598) (55.5244, 1.8598) (55.0767, 1.6694) (54.8915, 1.4842) knots 0 0 0 1 2 2 2
  spline S146 degree 2 poles (54.8915, 1.4842) (54.7114, 1.2938) (54.5261, 0.8358) (54.5004, 0.5322) knots 0 0 0 1 2 2 2
  line L102 (54.5004, 0.5322) -> (57.0167, 0.5322)
  spline S147 degree 2 poles (60.6806, -2.4884) (59.5382, -2.4884) (58.2826, -1.2071) (58.2826, -0.0236) knots 0 0 0 1 2 2 2
  spline S148 degree 2 poles (58.2826, -0.0236) (58.2826, 1.1394) (59.5022, 2.5185) (60.485, 2.5185) knots 0 0 0 1 2 2 2
  spline S149 degree 2 poles (60.485, 2.5185) (60.9276, 2.5185) (61.612, 2.2612) (61.8641, 1.9885) knots 0 0 0 1 2 2 2
  spline S150 degree 2 poles (61.8641, 1.9885) (62.1214, 1.7157) (62.3942, 0.9284) (62.3942, 0.3572) knots 0 0 0 1 2 2 2
  line L103 (62.3942, 0.3572) -> (62.3942, -0.0802)
  line L104 (62.3942, -0.0802) -> (59.0957, -0.0802)
  spline S151 degree 2 poles (59.0957, -0.0802) (59.0957, -0.9086) (59.9293, -1.7886) (60.6703, -1.7886) knots 0 0 0 1 2 2 2
  spline S152 degree 2 poles (60.6703, -1.7886) (60.9327, -1.7886) (61.4422, -1.6702) (61.648, -1.5776) knots 0 0 0 1 2 2 2
  spline S153 degree 2 poles (61.648, -1.5776) (61.8641, -1.4747) (62.1626, -1.2946) (62.2604, -1.2122) knots 0 0 0 1 2 2 2
  line L105 (62.2604, -1.2122) -> (62.3067, -1.2122)
  line L106 (62.3067, -1.2122) -> (62.3067, -2.087)
  spline S154 degree 2 poles (62.3067, -2.087) (62.1677, -2.1437) (61.7458, -2.3083) (61.5811, -2.3546) knots 0 0 0 1 2 2 2
  spline S155 degree 2 poles (61.5811, -2.3546) (61.3495, -2.4215) (60.9687, -2.4884) (60.6806, -2.4884) knots 0 0 0 1 2 2 2
  spline S156 degree 2 poles (61.612, 0.5322) (61.6017, 0.8564) (61.4679, 1.3298) (61.3392, 1.4893) knots 0 0 0 1 2 2 2
  spline S157 degree 2 poles (61.3392, 1.4893) (61.2003, 1.6694) (60.7629, 1.8598) (60.4387, 1.8598) knots 0 0 0 1 2 2 2
  spline S158 degree 2 poles (60.4387, 1.8598) (60.1197, 1.8598) (59.672, 1.6694) (59.4867, 1.4842) knots 0 0 0 1 2 2 2
  spline S159 degree 2 poles (59.4867, 1.4842) (59.3066, 1.2938) (59.1214, 0.8358) (59.0957, 0.5322) knots 0 0 0 1 2 2 2
  line L107 (59.0957, 0.5322) -> (61.612, 0.5322)
  line L108 (64.0254, -2.3804) -> (63.2226, -2.3804)
  line L109 (63.2226, -2.3804) -> (63.2226, 4.2527)
  line L110 (63.2226, 4.2527) -> (64.0254, 4.2527)
  line L111 (64.0254, 4.2527) -> (64.0254, -2.3804)
  spline S160 degree 2 poles (67.2724, -2.4884) (66.1301, -2.4884) (64.8745, -1.2071) (64.8745, -0.0236) knots 0 0 0 1 2 2 2
  spline S161 degree 2 poles (64.8745, -0.0236) (64.8745, 1.1394) (66.094, 2.5185) (67.0769, 2.5185) knots 0 0 0 1 2 2 2
  spline S162 degree 2 poles (67.0769, 2.5185) (67.5194, 2.5185) (68.2038, 2.2612) (68.456, 1.9885) knots 0 0 0 1 2 2 2
  spline S163 degree 2 poles (68.456, 1.9885) (68.7133, 1.7157) (68.986, 0.9284) (68.986, 0.3572) knots 0 0 0 1 2 2 2
  line L112 (68.986, 0.3572) -> (68.986, -0.0802)
  line L113 (68.986, -0.0802) -> (65.6875, -0.0802)
  spline S164 degree 2 poles (65.6875, -0.0802) (65.6875, -0.9086) (66.5211, -1.7886) (67.2621, -1.7886) knots 0 0 0 1 2 2 2
  spline S165 degree 2 poles (67.2621, -1.7886) (67.5246, -1.7886) (68.034, -1.6702) (68.2399, -1.5776) knots 0 0 0 1 2 2 2
  spline S166 degree 2 poles (68.2399, -1.5776) (68.456, -1.4747) (68.7544, -1.2946) (68.8522, -1.2122) knots 0 0 0 1 2 2 2
  line L114 (68.8522, -1.2122) -> (68.8985, -1.2122)
  line L115 (68.8985, -1.2122) -> (68.8985, -2.087)
  spline S167 degree 2 poles (68.8985, -2.087) (68.7596, -2.1437) (68.3376, -2.3083) (68.173, -2.3546) knots 0 0 0 1 2 2 2
  spline S168 degree 2 poles (68.173, -2.3546) (67.9414, -2.4215) (67.5606, -2.4884) (67.2724, -2.4884) knots 0 0 0 1 2 2 2
  spline S169 degree 2 poles (68.2038, 0.5322) (68.1935, 0.8564) (68.0598, 1.3298) (67.9311, 1.4893) knots 0 0 0 1 2 2 2
  spline S170 degree 2 poles (67.9311, 1.4893) (67.7922, 1.6694) (67.3548, 1.8598) (67.0306, 1.8598) knots 0 0 0 1 2 2 2
  spline S171 degree 2 poles (67.0306, 1.8598) (66.7115, 1.8598) (66.2638, 1.6694) (66.0786, 1.4842) knots 0 0 0 1 2 2 2
  spline S172 degree 2 poles (66.0786, 1.4842) (65.8985, 1.2938) (65.7132, 0.8358) (65.6875, 0.5322) knots 0 0 0 1 2 2 2
  line L116 (65.6875, 0.5322) -> (68.2038, 0.5322)
  line L117 (46.4548, -6.5165) -> (44.2678, -12.8665)
  line L118 (44.2678, -12.8665) -> (43.357, -12.8665)
  line L119 (43.357, -12.8665) -> (41.17, -6.5165)
  line L120 (41.17, -6.5165) -> (42.0757, -6.5165)
  line L121 (42.0757, -6.5165) -> (43.8356, -11.791)
  line L122 (43.8356, -11.791) -> (45.5955, -6.5165)
  line L123 (45.5955, -6.5165) -> (46.4548, -6.5165)
  spline S173 degree 2 poles (50.906, -9.6915) (50.906, -11.3999) (49.9129, -13.0003) (48.8785, -13.0003) knots 0 0 0 1 2 2 2
  spline S174 degree 2 poles (48.8785, -13.0003) (47.8288, -13.0003) (46.8459, -11.369) (46.8459, -9.6966) knots 0 0 0 1 2 2 2
  spline S175 degree 2 poles (46.8459, -9.6966) (46.8459, -7.9779) (47.8391, -6.3878) (48.8785, -6.3878) knots 0 0 0 1 2 2 2
  spline S176 degree 2 poles (48.8785, -6.3878) (49.9231, -6.3878) (50.906, -8.0345) (50.906, -9.6915) knots 0 0 0 1 2 2 2
  spline S177 degree 2 poles (49.8151, -11.6263) (49.9386, -11.3124) (50.0415, -10.345) (50.0415, -9.6915) knots 0 0 0 1 2 2 2
  spline S178 degree 2 poles (50.0415, -9.6915) (50.0415, -9.038) (49.9386, -8.0757) (49.8099, -7.7515) knots 0 0 0 1 2 2 2
  spline S179 degree 2 poles (49.8099, -7.7515) (49.6813, -7.4273) (49.2336, -7.0928) (48.8785, -7.0928) knots 0 0 0 1 2 2 2
  spline S180 degree 2 poles (48.8785, -7.0928) (48.5235, -7.0928) (48.0655, -7.4273) (47.9317, -7.7618) knots 0 0 0 1 2 2 2
  spline S181 degree 2 poles (47.9317, -7.7618) (47.803, -8.086) (47.7104, -9.074) (47.7104, -9.6966) knots 0 0 0 1 2 2 2
  spline S182 degree 2 poles (47.7104, -9.6966) (47.7104, -10.3656) (47.7928, -11.261) (47.9265, -11.6109) knots 0 0 0 1 2 2 2
  spline S183 degree 2 poles (47.9265, -11.6109) (48.05, -11.9402) (48.508, -12.2953) (48.8785, -12.2953) knots 0 0 0 1 2 2 2
  spline S184 degree 2 poles (48.8785, -12.2953) (49.2285, -12.2953) (49.6864, -11.9608) (49.8151, -11.6263) knots 0 0 0 1 2 2 2
  line L124 (55.6351, -12.8665) -> (51.7191, -12.8665)
  line L125 (51.7191, -12.8665) -> (51.7191, -11.966)
  spline S185 degree 2 poles (51.7191, -11.966) (52.141, -11.5697) (52.8923, -10.8339) (53.2525, -10.4376) knots 0 0 0 1 2 2 2
  spline S186 degree 2 poles (53.2525, -10.4376) (53.9781, -9.64) (54.5081, -8.6829) (54.5081, -8.1735) knots 0 0 0 1 2 2 2
  spline S187 degree 2 poles (54.5081, -8.1735) (54.5081, -7.9059) (54.3434, -7.5045) (54.1942, -7.3759) knots 0 0 0 1 2 2 2
  spline S188 degree 2 poles (54.1942, -7.3759) (54.045, -7.2472) (53.6539, -7.1186) (53.4172, -7.1186) knots 0 0 0 1 2 2 2
  spline S189 degree 2 poles (53.4172, -7.1186) (53.1908, -7.1186) (52.7276, -7.2318) (52.5167, -7.3192) knots 0 0 0 1 2 2 2
  spline S190 degree 2 poles (52.5167, -7.3192) (52.3366, -7.3913) (52.0021, -7.5971) (51.8992, -7.6692) knots 0 0 0 1 2 2 2
  line L126 (51.8992, -7.6692) -> (51.8528, -7.6692)
  line L127 (51.8528, -7.6692) -> (51.8528, -6.7635)
  spline S191 degree 2 poles (51.8528, -6.7635) (52.1153, -6.6348) (53.057, -6.3827) (53.4789, -6.3827) knots 0 0 0 1 2 2 2
  spline S192 degree 2 poles (53.4789, -6.3827) (54.3692, -6.3827) (55.3726, -7.3244) (55.3726, -8.1271) knots 0 0 0 1 2 2 2
  spline S193 degree 2 poles (55.3726, -8.1271) (55.3726, -8.5028) (55.1977, -9.1306) (55.0433, -9.3982) knots 0 0 0 1 2 2 2
  spline S194 degree 2 poles (55.0433, -9.3982) (54.8889, -9.6761) (54.4412, -10.2215) (54.1942, -10.484) knots 0 0 0 1 2 2 2
  spline S195 degree 2 poles (54.1942, -10.484) (53.7928, -10.9214) (52.81, -11.8579) (52.5167, -12.1306) knots 0 0 0 1 2 2 2
  line L128 (52.5167, -12.1306) -> (55.6351, -12.1306)
  line L129 (55.6351, -12.1306) -> (55.6351, -12.8665)
  point P0 (48.5775, 0)
  constraints: 2 end point, 2 horizontal
extrude "Extrusion11" cut sketch "Sketch14" against normal blind 3.175
equation "\"majorPartWidth\" = holeForPiCaseWidth + 2 * minWallThickness"
equation "\"majorPartHeight\" = lightRingHoleExteriorDiam + 2 * minWallThickness"
equation "\"majorPartDepth\" = holeForPiCaseDepth + minWallThickness"
equation "\"holeForPiCaseWidth\" = piCaseWidth + 2 * caseGap"
equation "\"holeForPiCaseHeight\" = piCaseHeight + 2 * caseGap"
equation "\"holeForPiCaseDepth\" = PiCaseDepth + depthForLightRing"
equation "\"lightRingHoleExteriorDiam\" = lightRingExteriorDiam + lightRingEdgeSpacing"
equation "\"lightRingHoleInteriorDiam\" = lightRingInterorDiam - lightRingEdgeSpacing"
equation "\"d13\" = holeForLightRingWires"
equation "\"baseWidth\" = majorPartWidth"
equation "\"y\" = 0.5 * PiCaseDepth + depthForLightRing"
equation "\"Y\" = 0.5 * majorPartWidth"
equation "\"minWallThickness\" = 6.35"
equation "\"lightRingEdgeSpacing\" = 3"
equation "\"lightRingExteriorDiam\" = 60"
equation "\"lightRingInterorDiam\" = 40"
equation "\"caseGap\" = 2.54"
equation "\"piCaseWidth\" = 79.375"
equation "\"piCaseHeight\" = 38.1"
equation "\"PiCaseDepth\" = 15.875"
equation "\"depthForLightRing\" = 2.5"
body "Solid1"
